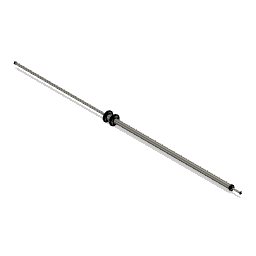
deuterium compression device v6 (Autodesk Fusion 360 design; units mm, degrees)
Autodesk Fusion 360 part; units mm, degrees
note: some values were not read from the file. Set by a fixed rule: which sketch regions a step uses.
sketch "Sketch1" plane through (0, 0, 0) normal (0, 1, 0) x (1, 0, 0)
  line L0 (-500, 0) -> (-500, 4)
  line L1 (-500, 4) -> (0, 4)
  line L2 (0, 4) -> (0, 0)
  line L3 (0, 0) -> (-500, 0)
  line L4 (0, 4) -> (400, 4)
  line L5 (400, 4) -> (400, 8)
  line L6 (400, 8) -> (-84.4, 8)
  line L7 (-84.4, 8) -> (-84.4, 7.5)
  line L8 (-84.4, 7.5) -> (-88.9, 7.5)
  line L9 (-88.9, 7.5) -> (-88.9, 7.15)
  line L10 (-88.9, 7.15) -> (-90, 7.15)
  line L11 (-90, 7.15) -> (-90, 7.5)
  line L12 (-90, 7.5) -> (-95, 7.5)
  line L13 (-95, 7.5) -> (-95, 7)
  line L14 (-95, 7) -> (-100, 7)
  line L15 (-100, 7) -> (-100, 4)
  line L16 (-95, 7.5) -> (-95, 10)
  line L17 (-95, 10) -> (-112, 10)
  line L18 (-112, 10) -> (-112, 4)
  line L19 (-107, 4) -> (-107, 7)
  line L20 (-107, 7) -> (-100, 7)
  line L21 (-112, 10) -> (-112, 17)
  line L22 (-112, 17) -> (-116, 17)
  line L23 (-116, 17) -> (-116, 4)
  line L24 (-88.9, 7.5) -> (-88.9, 17)
  line L25 (-88.9, 17) -> (-84.9, 17)
  line L26 (-84.9, 17) -> (-84.9, 7.5)
  line L27 (-116, 13) -> (-112, 13) construction
  line L28 (400, 8) -> (400, 3)
  line L29 (400, 3) -> (404, 3)
  line L30 (404, 3) -> (404, 8)
  line L31 (404, 8) -> (400, 8)
  line L32 (400, 3) -> (400, 1)
  line L33 (400, 1) -> (440, 1)
  line L34 (440, 1) -> (440, 3)
  line L35 (440, 3) -> (400, 3)
  dimension "d1" = 4
  dimension "d2" = 500
  dimension "d4" = 7.15
  dimension "d5" = 8
  dimension "d6" = 7
  dimension "d7" = 7.5
  dimension "d8" = 5
  dimension "d9" = 5
  dimension "d10" = 1.1
  dimension "d11" = 4.5
  dimension "d12" = 500
  dimension "d13" = 100
  dimension "d14" = 7
  dimension "d15" = 5
  dimension "d16" = 10
  dimension "d17" = 4
  dimension "d18" = 4
  dimension "d19" = 3
  dimension "d33" = 4
  dimension "d34" = 3
  dimension "d40" = 40
  dimension "d41" = 2
  constraint vertical L0
  constraint perpendicular L0 L1
  constraint perpendicular L1 L2
  constraint perpendicular L0 L3
  constraint perpendicular L2 L4
  constraint perpendicular L4 L5
  constraint perpendicular L5 L6
  constraint perpendicular L6 L7
  constraint perpendicular L7 L8
  constraint perpendicular L8 L9
  constraint perpendicular L9 L10
  constraint perpendicular L10 L11
  constraint perpendicular L11 L12
  constraint perpendicular L12 L13
  constraint perpendicular L13 L14
  constraint coincident L1 L15.end
  constraint perpendicular L1 L15
  constraint coincident L2.end L3
  constraint collinear L8 L12
  constraint coincident L2.end L3.start
  constraint perpendicular L12 L16
  constraint perpendicular L16 L17
  constraint perpendicular L1 L18
  constraint coincident L1 L18.end
  constraint coincident L1 L19.start
  constraint perpendicular L14 L19
  constraint perpendicular L15 L20
  constraint perpendicular L17 L21
  constraint perpendicular L21 L22
  constraint coincident L1 L23.end
  constraint perpendicular L1 L23
  constraint perpendicular L8 L24
  constraint perpendicular L9 L25
  constraint coincident L8 L26.end
  constraint perpendicular L8 L26
  constraint collinear L22 L25
  constraint equal L22 L25
  constraint coincident L23 L27.start
  constraint coincident L21 L27.end
  constraint perpendicular L21 L27
  constraint perpendicular L6 L28
  constraint perpendicular L5 L29
  constraint perpendicular L6 L30
  constraint perpendicular L28 L31
  constraint perpendicular L29 L32
  constraint perpendicular L32 L33
  constraint perpendicular L33 L34
  constraint perpendicular L28 L35
  measures "d1" distance of L0.start L0.end
  measures "d2" distance of L0.end L1.end
  measures "d4" distance of L3 L10
  measures "d5" distance of L3 L6
  measures "d6" distance of L3 L14
  measures "d7" distance of L3 L12
  measures "d8" distance of L13.end L14.end
  measures "d9" distance of L11.end L12.end
  measures "d10" distance of L9.end L10.end
  measures "d11" distance of L7.end L8.end
  measures "d12" distance of L5 L15
  measures "d13" distance of L2 L15
  measures "d14" distance of L15 L19
  measures "d15" distance of L18 L19
  measures "d16" distance of L3 L17
  measures "d17" distance of L21.end L22.end
  measures "d18" distance of L22 L27
  measures "d19" distance of L17 L27
  measures "d33" distance of L28.end L29.end
  measures "d34" distance of L2.end L29
  measures "d40" distance of L32.end L33.end
  measures "d41" distance of L33 L35
revolve "Revolve1" add sketch "Sketch1" angle 360 about axis through (0, 0, 0) along (-1, 0, 0) contours L0 L1 L2 L3 makes body 1
revolve "Revolve2" add sketch "Sketch1" angle 360 about axis through (1.75, 0, 0) along (1, 0, 0) separate body contours L1 L4 L5 L6 L7 L8 L9 L10 L11 L12 L13 L14 L15 L28 makes body 2
revolve "Revolve3" add sketch "Sketch1" angle 360 about axis through (-500, 0, 0) along (1, 0, 0) separate body contours L1 L13 L14 L16 L17 L18 L19 L20 makes body 3
revolve "Revolve4" add sketch "Sketch1" angle 360 about axis through (400, 0, 0) along (-1, 0, 0) separate body contours L8 L24 L25 L26 makes body 4
revolve "Revolve5" add sketch "Sketch1" angle 360 about axis through (-500, 0, 0) along (1, 0, 0) separate body contours L1 L18 L21 L22 L23 makes body 5
sketch "Sketch2" plane through (-116, 0, 0) normal (-1, 0, 0) x (0, 0, 1)
  circle A0 centre (0, 0) radius 4
  circle A1 centre (0, 0) radius 17
  point P0 (-13, 0)
hole "Hole1" at (-116, 0, -13) direction (1, 0, 0) diameter 6.6 depth 45 tip angle 118 bodies 4 5
pattern_circular "C-Pattern1" count 3 over 360 about axis through (-84.4, 0, 0) along (1, 0, 0) of "Hole1"
chamfer "Chamfer1" distance 0.5 angle 45 2 edges at (-112, -3.6162, 9.3233) (-95, -3.6162, 9.3233) on bodies 3
revolve "Drehen6" add sketch "Sketch1" angle 360 about axis through (400, 0, 0) along (-1, 0, 0) separate body contours L5 L28 L29 L30 L31 L35 makes body 6
revolve "Drehen7" add sketch "Sketch1" angle 360 about axis through (400, 0, 0) along (-1, 0, 0) separate body contours L29 L32 L33 L34 L35 makes body 7
chamfer "Fase3" distance 0.5 angle 45 1 edges at (400, -2.8929, 7.4586) on bodies 6
equation "d4 = ( 14.3 / 2 ) * 1 mm"
named bodies: "Kolbenstange", "Rohr", "Ueberwurf", "Schraubplatte Rohr", "Schraubplatte Kolben", "Endstopfen", "Rohranbindung"
